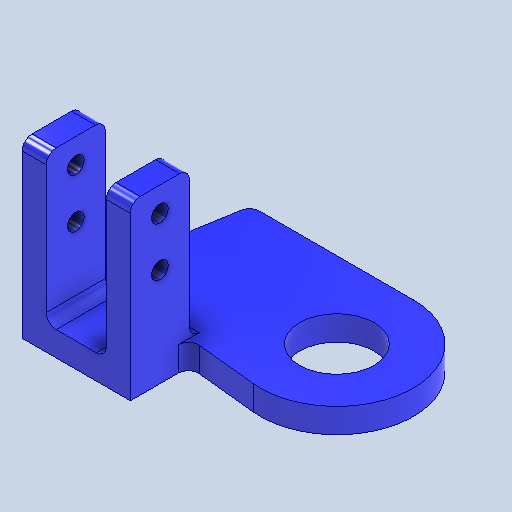
# Autodesk Inventor part: roller-hand-v1-3DP-bearing-r-side
Saved by Autodesk Inventor 2025.1 (Build 291241000, 241)
## iProperties
Created: 2024-10-01
Part Number: roller-hand-v1-3DP-bearing-r-side
Material: ABS プラスチック
Document SubType Name: Modeling
Designer: haruy
Density: 1.06 g/cm^3
Appearance: 青 - 壁塗料 - 光沢
Author: haruy
Autodesk Inventor part; units mm, degrees
ref_plane "YZ Plane" through (0, 0, 0) normal (1, 0, 0) x (0, 1, 0)
ref_plane "XZ Plane" through (0, 0, 0) normal (0, 1, 0) x (-1, 0, 0)
ref_plane "XY Plane" through (0, 0, 0) normal (0, 0, 1) x (1, 0, 0)
derived "roller-hand-v1-Sketch-Base.ipt"
sketch "スケッチ1" plane through (0, 0, 0) normal (1, 0, 0) x (0, 1, 0)
  circle A0 centre (0, 0) radius 600
  circle A1 centre (0, 0) radius 400
  circle A2 centre (429.926, 0) radius 122.5
  line L0 (-287.7615, 277.8368) -> (287.7615, 277.8368)
  line L1 (287.7615, 277.8368) -> (287.7615, -277.8368)
  line L2 (287.7615, -277.8368) -> (-287.7615, -277.8368)
  line L3 (-287.7615, -277.8368) -> (-287.7615, 277.8368)
  line L4 (-287.7615, 277.8368) -> (287.7615, -277.8368) construction
  line L5 (287.7615, 277.8368) -> (-287.7615, -277.8368) construction
  line L6 (565.0687, 140.5) -> (285.0687, 140.5)
  line L7 (285.0687, 140.5) -> (285.0687, 122.5)
  line L8 (285.0687, 122.5) -> (565.0687, 122.5)
  line L9 (565.0687, 122.5) -> (565.0687, 140.5)
  line L10 (565.0687, -122.5) -> (285.0687, -122.5)
  line L11 (285.0687, -122.5) -> (285.0687, -140.5)
  line L12 (285.0687, -140.5) -> (565.0687, -140.5)
  line L13 (565.0687, -140.5) -> (565.0687, -122.5)
  line L14 (270.0687, 141.5) -> (242.6687, 141.5)
  line L15 (242.6687, 141.5) -> (242.6687, 121.5)
  line L16 (242.6687, 121.5) -> (270.0687, 121.5)
  line L17 (270.0687, 121.5) -> (270.0687, 141.5)
  line L18 (231.8687, 147.5) -> (160.1687, 147.5)
  line L19 (160.1687, 147.5) -> (160.1687, 115.5)
  line L20 (160.1687, 115.5) -> (231.8687, 115.5)
  line L21 (231.8687, 115.5) -> (231.8687, 147.5)
  line L22 (231.8687, 141.5) -> (235.8687, 141.5)
  line L23 (235.8687, 141.5) -> (235.8687, 121.5)
  line L24 (235.8687, 121.5) -> (231.8687, 121.5)
  line L25 (231.8687, 121.5) -> (231.8687, 141.5)
  line L26 (235.8687, 134.5) -> (250.6687, 134.5)
  line L27 (250.6687, 134.5) -> (250.6687, 128.5)
  line L28 (250.6687, 128.5) -> (235.8687, 128.5)
  line L29 (235.8687, 128.5) -> (235.8687, 134.5)
  line L30 (300.0687, 136.5) -> (262.0687, 136.5)
  line L31 (262.0687, 136.5) -> (262.0687, 126.5)
  line L32 (262.0687, 126.5) -> (300.0687, 126.5)
  line L33 (300.0687, 126.5) -> (300.0687, 136.5)
  line L34 (280.0687, 145.0404) -> (275.0687, 145.0404)
  line L35 (275.0687, 145.0404) -> (275.0687, 91.5358)
  line L36 (275.0687, 91.5358) -> (280.0687, 91.5358)
  line L37 (280.0687, 91.5358) -> (280.0687, 145.0404)
  line L38 (275.0687, 145.5) -> (263.0687, 145.5)
  line L39 (263.0687, 145.5) -> (263.0687, -145.5)
  line L40 (263.0687, -145.5) -> (275.0687, -145.5)
  line L41 (275.0687, -145.5) -> (275.0687, 145.5)
  line L42 (565.0687, 157.5) -> (263.0687, 157.5)
  line L43 (263.0687, 157.5) -> (263.0687, 145.5)
  line L44 (263.0687, 145.5) -> (565.0687, 145.5)
  line L45 (565.0687, 145.5) -> (565.0687, 157.5)
  line L46 (575.0687, 157.5) -> (570.0687, 157.5)
  line L47 (570.0687, 157.5) -> (570.0687, 122.5)
  line L48 (570.0687, 122.5) -> (575.0687, 122.5)
  line L49 (575.0687, 122.5) -> (575.0687, 157.5)
  line L50 (565.0687, -145.5) -> (263.0687, -145.5)
  line L51 (263.0687, -145.5) -> (263.0687, -157.5)
  line L52 (263.0687, -157.5) -> (565.0687, -157.5)
  line L53 (565.0687, -157.5) -> (565.0687, -145.5)
  circle A3 centre (269.0687, 140.5) radius 1.7
  circle A4 centre (269.0687, 130.5) radius 1.7
  circle A5 centre (269.0687, 151.5) radius 1.7
  circle A6 centre (286.0687, 151.5) radius 1.7
  circle A7 centre (555.0687, 151.5) radius 1.5
  circle A8 centre (545.0687, 151.5) radius 1.5
  line L54 (0, 0) -> (429.926, 0)
  circle A9 centre (555.0687, -151.5) radius 1.5
  circle A10 centre (545.0687, -151.5) radius 1.5
  circle A11 centre (269.0687, -130.5) radius 1.7
  circle A12 centre (269.0687, -140.5) radius 1.7
  circle A13 centre (269.0687, -151.5) radius 1.7
  circle A14 centre (286.0687, -151.5) radius 1.7
sketch "スケッチ2" plane through (0, 0, 0) normal (0, 1, 0) x (-1, 0, 0)
  circle A0 centre (0, 0) radius 9
  line L0 (33, 14) -> (21, 14)
  line L1 (21, 14) -> (21, -141.0479)
  line L2 (21, -141.0479) -> (33, -141.0479)
  line L3 (33, -141.0479) -> (33, 14)
  line L4 (33, 26) -> (21, 26)
  line L5 (21, 26) -> (21, 14)
  line L6 (21, 14) -> (33, 14)
  line L7 (33, 14) -> (33, 26)
  circle A1 centre (0, 0) radius 16
  circle A2 centre (0, 0) radius 21
  circle A3 centre (14.8492, 14.8492) radius 1.7
  circle A4 centre (-14.8492, 14.8492) radius 1.7
  circle A5 centre (-14.8492, -14.8492) radius 1.7
  circle A6 centre (14.8492, -14.8492) radius 1.7
  circle A7 centre (14.8492, 14.8492) radius 4.7
  circle A8 centre (14.8492, -14.8492) radius 4.7
  circle A9 centre (-14.8492, 14.8492) radius 4.7
  circle A10 centre (-14.8492, -14.8492) radius 4.7
  circle A11 centre (27, 4) radius 1.7
  circle A12 centre (27, -6) radius 1.7
  line L8 (21, 14) -> (18.7936, 17.4051)
  line L9 (14.8492, 19.5492) -> (-14.8492, 19.5492)
  line L10 (-19.5492, 14.8492) -> (-19.5492, -14.8492)
  line L11 (-14.8492, -19.5492) -> (14.8492, -19.5492)
  line L12 (33, -19.5492) -> (21, -19.5492)
  line L13 (21, -19.5492) -> (14.8492, -19.5492)
  circle A13 centre (0, 0) radius 7.55
  circle A14 centre (14.8492, 14.8492) radius 3
  circle A15 centre (14.8492, -14.8492) radius 3
  circle A16 centre (-14.8492, 14.8492) radius 3
  circle A17 centre (-14.8492, -14.8492) radius 3
  circle A18 centre (0, 0) radius 15.55
  line L14 (0, -15.55) -> (33, -15.55)
  line L15 (33, 26) -> (38, 26)
  line L16 (38, 26) -> (38, 14)
  line L17 (38, 14) -> (33, 14)
  line L18 (33, 14) -> (33, 26)
  line L19 (21, 26) -> (16, 26)
  line L20 (16, 26) -> (16, 14)
  line L21 (16, 14) -> (21, 14)
  line L22 (21, 14) -> (21, 26)
  line L23 (38, 14) -> (33, -15.55)
  line L24 (16, 14) -> (1.5765, 15.4699)
  line L25 (38, 26) -> (33.1, 26)
  line L26 (33.1, 26) -> (33.1, 14)
  line L27 (33.1, 14) -> (38, 14)
  line L28 (38, 14) -> (38, 26)
  line L29 (16, 26) -> (20.9, 26)
  line L30 (20.9, 26) -> (20.9, 14)
  line L31 (20.9, 14) -> (16, 14)
  line L32 (16, 14) -> (16, 26)
  point P0 (0, 21)
  point P1 (20.9, 14.1543)
  dimension "d1" = 8
  dimension "d2" = 5
  dimension "d3" = 12
  dimension "d4" = 5
  dimension "d5" = 12
  dimension "d6" = 4.9
  dimension "d7" = 12
  dimension "d8" = 4.9
  dimension "d9" = 12
  measures "d1" radial gap between concentric circles of A13 A18
  measures "d2" distance of L16.end L17.end
  measures "d3" distance of L15.end L16.end
  measures "d4" distance of L21.end L20.end
  measures "d5" distance of L20.end L19.end
  measures "d6" distance of L27.end L26.end
  measures "d7" distance of L26.end L25.end
  measures "d8" distance of L30.end L31.end
  measures "d9" distance of L29.end L30.end
extrude "押し出し1" add sketch "スケッチ2" against normal blind 5 contours A0 | L3 L14 L1 L0 | L17 L23 L3 | L0 L5 L4 L7 | L7 L15 L26 L17 | L8 L30 L19 L5 | L21 L30 L8 | L1 A2 A7 L21 | L26 L15 L16 L17 | A2 A8 L14 A1 L24 A7 | L1 L14 A8 A2 | L30 L21 A7 L8 | L8 A7 L20 L19 L30 | A7 L24 A14 A2 | A2 A14 L21 A7 | A8 L14 A15 A2 | A2 A15 L14 A8 | A7 L21 A14 L20 | A14 L24 A3 A2 | A2 A3 L21 A14 | A15 L14 A6 A2 | A2 A6 L14 A15 | L21 A3 L20 A14 | A3 L24 A2 | A2 L24 L21 A3 | A1 L14 A18 L24 | A6 L14 A2 | A2 L14 A6 | L21 L20 A3 | A18 | A11 | A12 picked at (16.0287, 10.9139) picked at (18.9204, -14.288) picked at (16.0636, -10.9231) picked at (14.6165, 12.3107) picked at (17.381, -14.5205) picked at (15.7065, -12.4474) picked at (14.0998, 14.0753) picked at (4.0605, 15.0613) picked at (15.0942, -15.3424) picked at (14.7348, -14.1872)
extrude "押し出し2" add sketch "スケッチ2" along normal blind 30 contours L26 L15 L16 L17 | L30 L21 A7 L8 | L8 A7 L20 L19 L30 | A7 L21 A14 L20 | L21 A3 L20 A14 | L21 L20 A3
fillet "フィレット1" radius 2 11 edges at (-20.9, 0, 20) (-18.45, 0, 14) (-33.1, 0, 20) (-35.55, 0, 14) (-33, -2.5, -15.55) (-38, -2.5, 14) (-35.55, 30, 26) (-35.55, 30, 14) (-16, -2.5, 14) (-18.45, 30, 26) (-18.45, 30, 14)
sketch "スケッチ3" plane through (-38, -5, 14.168) normal (-1, 0, 0) x (0, 0, 1)
  line L0 (1.832, 35) -> (9.832, 35) projected
  line L1 (11.832, 0) -> (11.832, 33) projected
  point P0 (-14.168, 5)
  point P1 (5.832, 30)
  point P2 (5.832, 20)
  dimension "d15" = 5
  dimension "d17" = 10
  dimension "d18" = 6
  dimension "d19" = 6
  measures "d15" distance from line of point (5.832, 30) L0
  measures "d17" distance of point (5.832, 30) point (5.832, 20)
  measures "d18" distance from line of point (5.832, 30) L1
  measures "d19" distance from line of L1 point (5.832, 20)
hole "穴1" at (-38, 25, 20) at (-38, 15, 20) direction (1, 0, 0) diameter 3.4 end through all
equation "\"d19\" = d18"
